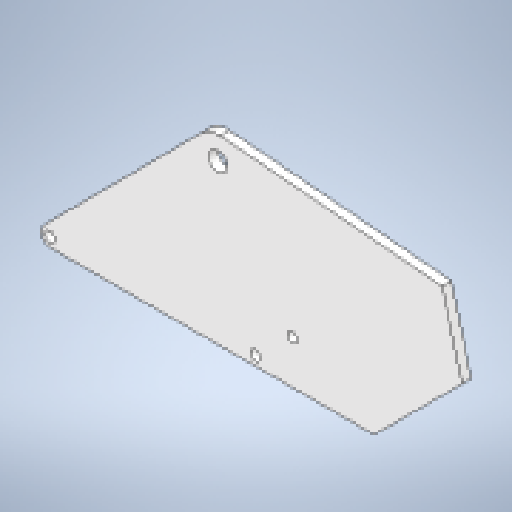
# Autodesk Inventor part: Uprights
Saved by Autodesk Inventor 2023.2 (Build 272271000, 271)
## iProperties
Created: 2024-01-11
Part Number: Uprights
Material: UHMW, White
Document SubType Name: Modeling
Designer: Nathan Cai
Mass: 18.9298 g
Surface Area: 139.502 cm^2
Volume: 20.1381 cm^3
Density: 0.94 g/cm^3
Appearance: Smooth - White
Author: Nathan Cai
Autodesk Inventor part; units mm, degrees
ref_plane "YZ Plane" through (0, 0, 0) normal (1, 0, 0) x (0, 1, 0)
ref_plane "XZ Plane" through (0, 0, 0) normal (0, 1, 0) x (-1, 0, 0)
ref_plane "XY Plane" through (0, 0, 0) normal (0, 0, 1) x (1, 0, 0)
sketch "Sketch2" plane through (0, 0, 0) normal (0, 0, 1) x (1, 0, 0)
  circle A0 centre (0, 0) radius 3.175
  circle A1 centre (0, 0) radius 7.9375
  line L0 (-24.9815, -53.975) -> (30.0677, -53.975)
  line L1 (-24.9815, -53.975) -> (-36.2864, -11.7845)
  line L2 (-36.2864, -11.7845) -> (-3.9687, 6.8741)
  line L3 (20.5427, -47.625) -> (-13.5349, -47.625)
  line L4 (-13.5349, -47.625) -> (-22.3476, -14.7355)
  line L5 (-22.3476, -14.7355) -> (-5.9414, -5.2634)
  line L6 (-18.1512, -42.6641) -> (-23.9035, -21.1964) construction
  line L7 (-23.9035, -21.1964) -> (-30.0371, -22.8399) construction
  line L8 (-30.0371, -22.8399) -> (-24.2848, -44.3076) construction
  line L9 (-24.2848, -44.3076) -> (-18.1512, -42.6641) construction
  line L10 (-18.1512, -42.6641) -> (-30.0371, -22.8399) construction
  line L11 (-23.9035, -21.1964) -> (-24.2848, -44.3076) construction
  circle A2 centre (-30.0371, -22.8399) radius 1.7526
  circle A3 centre (-24.2848, -44.3076) radius 1.7526
  circle A4 centre (-21.0273, -31.9303) radius 2
  line L12 (25.3052, -45.5804) -> (25.3052, -53.975) construction
  circle A5 centre (25.3052, -39.2375) radius 1.7526
  line L13 (0, 0) -> (-58.6646, -15.7191) construction
  line L14 (-24.0941, -32.752) -> (-30.6681, -8.2175) construction
  circle A6 centre (25.3052, -39.2375) radius 4.7625
  line L15 (30.0677, -39.2375) -> (30.0677, -53.975)
  line L16 (20.5427, -39.2375) -> (20.5427, -47.625)
  line L17 (-30.2278, -34.3955) -> (-17.9605, -31.1085) construction
  circle A7 centre (-9.9632, -48.6877) radius 1.7526
  line L18 (-9.9632, -48.6877) -> (-25.2973, -52.7964) construction
  line L19 (25.3052, -39.2375) -> (24.0725, -34.6373) construction
  line L20 (-9.9632, -48.6877) -> (-10.4168, -46.9948) construction
  circle A8 centre (25.3052, -39.2375) radius 1.7526
  circle A9 centre (25.3052, -39.2375) radius 4.7625
  line L21 (16.8164, -38.2251) -> (8.188, -6.0235)
  line L22 (8.188, -6.0235) -> (-22.4801, -14.241) construction
  line L23 (-22.4801, -14.241) -> (-13.8518, -46.4426) construction
  line L24 (-13.8518, -46.4426) -> (16.8164, -38.2251)
  line L25 (16.8164, -38.2251) -> (-22.4801, -14.241) construction
  line L26 (8.188, -6.0235) -> (-13.8518, -46.4426) construction
  line L27 (6.9477, 3.8384) -> (29.4738, -36.9345)
  line L28 (2.0544, -7.667) -> (8.188, -6.0235)
  circle A10 centre (-9.9632, -48.6877) radius 4.7625 construction
  line L29 (26.5378, -43.8377) -> (-11.2949, -53.975)
  line L30 (76.2, 1.3012) -> (0.6918, 7.9073)
  line L31 (83.0059, -24.0988) -> (76.2, 1.3012)
  circle A11 centre (-57.15, -50.8) radius 1.7526
  circle A12 centre (-57.15, -50.8) radius 3.175
  line L32 (-57.15, -53.975) -> (-24.9815, -53.975)
  line L33 (-5.6327, 5.5926) -> (-59.4031, -48.563)
  circle A13 centre (12.7, -50.8) radius 1.7526
  line L34 (83.0059, -24.0988) -> (53.1297, -53.975)
  line L35 (53.1297, -53.975) -> (30.0677, -53.975)
  point P0 (7.667, 2.0544)
  point P1 (0.4795, -7.923)
  point P2 (-24.0941, -32.752)
  point P3 (-2.8319, -26.2331)
  point P4 (-2.8319, -26.2331)
  point P5 (-11.2949, -53.975)
  point P6 (-12.1309, -47.625)
  point P7 (-13.8518, -46.4426)
  point P8 (27.0578, -39.2375)
  point P9 (28.5531, -38.4633)
  point P10 (26.5378, -43.8377)
  point P11 (29.4738, -36.9345)
  dimension "d7" = 15.875
  dimension "d40" = 3.5052
  dimension "d6" = 6.35
  dimension "d15" = 105
  dimension "d17" = 105
  dimension "d19" = 9.525
  dimension "d20" = 12.7
  dimension "d24" = 22.225
  dimension "d25" = 6.35
  dimension "d26" = 3.5052
  dimension "d27" = 3.5052
  dimension "d28" = 4
  dimension "d29" = 6.35
  dimension "d33" = 3.5052
  dimension "d35" = 31.75
  dimension "d37" = 9.525
  dimension "d38" = 25.4
  dimension "d39" = 53.975
  dimension "d41" = 44.45
  dimension "d43" = 36.5125
  dimension "d48" = 22.225
  dimension "d49" = 3.5052
  dimension "d51" = 9.525
  dimension "d52" = 31.75
  dimension "d53" = 33.3375
  dimension "d54" = 9.525
  dimension "d56" = 145
  dimension "d58" = 110
  dimension "d60" = 76.2
  dimension "d61" = 25.4
  dimension "d63" = 3.5052
  dimension "d64" = 6.35
  dimension "d65" = 57.15
  dimension "d66" = 3.5052
  dimension "d67" = 3.175
  dimension "d69" = 69.85
  dimension "d70" = 135
  constraints: 72 end point, 12 centre point, 12 point on line, 10 perpendicular, 8 coincident, 8 midpoint, 8 point on circle, 7 parallel, 7 tangent, 2 collinear, 2 horizontal, 1 concentric, 18 other
  measures "d6" diameter of A0
  measures "d15" angle of L0 L1
  measures "d17" angle of L2 L1
  measures "d19" distance between parallel lines of L2 L5
  measures "d20" distance between parallel lines of L1 L4
  measures "d24" distance of L6.start L6.end
  measures "d25" distance of L7.end L6.end
  measures "d26" diameter of A2
  measures "d27" diameter of A3
  measures "d28" diameter of A4
  measures "d29" distance between parallel lines of L0 L3
  measures "d33" diameter of A5
  measures "d35" distance from line of point (0, 0) L14
  measures "d37" diameter of A6
  measures "d38" distance between parallel lines of L13 L17
  measures "d39" distance from line of L0 point (0, 0)
  measures "d41" distance between parallel lines of L13 L18
  measures "d43" distance from line of L18.start L19
  measures "d48" distance from line of point (0, 0) L20
  measures "d49" diameter of A8
  measures "d51" diameter of A9
  measures "d52" distance between parallel lines of L21 L23
  measures "d53" distance between parallel lines of L24 L22
  measures "d54" diameter of A10
  measures "d56" angle of L2 L30
  measures "d58" angle of L30 L31
  measures "d60" horizontal distance of L13.start L30.start
  measures "d61" vertical distance of L30.start L31.start
  measures "d63" diameter of A11
  measures "d64" diameter of A12
  measures "d65" horizontal distance of L13.start A12.centre
  measures "d66" diameter of A13
  measures "d67" distance from line of L0 A13.centre
  measures "d69" distance of A11.centre A13.centre
  measures "d70" angle of L35 L34
extrude "Extrusion2" add sketch "Sketch2" along normal blind 3.175 contours A1 | A1 L27 A6 L16 L29 L3 A7 L4 L24 L21 L28 | A1 L30 L31 L34 L35 L15 A6 L27 | L28 L21 L24 L4 L5 A1 | A6 | L5 L4 L3 A7 L29 L0 L1 L33 A1 | L15 L0 L29 L3 L16 A6 | A6 L29 L16 | L16 L3 L29 | L1 L32 A12 L33 | A12 | A7 L3 | L3 A7 | A2 | A3 | A4
equation "\"d26\" = d33"
equation "\"d27\" = d33"
body "Solid2"
